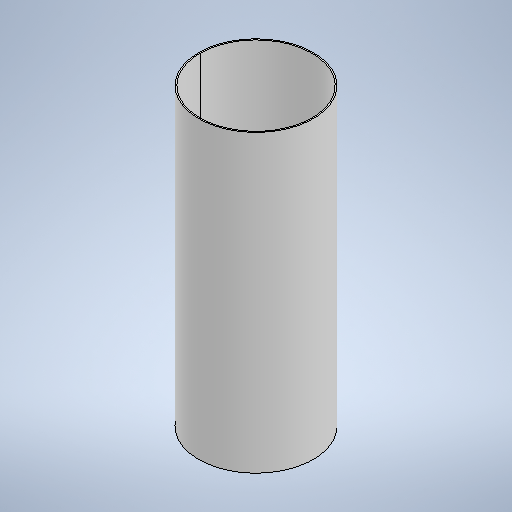
# Autodesk Inventor part: TZS 1291 accses hatch shell
Saved by Autodesk Inventor 2025 (Build 290162010, 162A)
## iProperties
Created: 2025-02-12
Part Number: TZS 1291 accses hatch shell
Material: Steel
Document SubType Name: Sheet Metal
Designer: admin
Mass: 13177.4 g
Surface Area: 5813.4 cm^2
Volume: 1678.65 cm^3
Density: 7.85 g/cm^3
Flat Pattern Width: 136 cm
Flat Pattern Length: 163.719 cm
Flat Pattern Area: 22265.8 cm^2
Sheet Metal Rule: Default_mm
Sheet Metal Width: 1360,000 mm
Sheet Metal Length: 1637,195 mm
Sheet Metal Area: 2226584,542 mm^2
Appearance: Default
Author: pokla
Autodesk Inventor part; units mm, degrees
ref_plane "YZ Plane" through (0, 0, 0) normal (1, 0, 0) x (0, 1, 0)
ref_plane "XZ Plane" through (0, 0, 0) normal (0, 1, 0) x (-1, 0, 0)
ref_plane "XY Plane" through (0, 0, 0) normal (0, 0, 1) x (1, 0, 0)
sketch "Sketch1" plane through (0, 0, 0) normal (0, 1, 0) x (-1, 0, 0)
  line L0 (258, 1360) -> (258, 0)
  line L1 (258, 0) -> (264, 0)
  line L2 (0, 0) -> (0, 109.131)
  line L3 (258, 1360) -> (264, 1360)
  line L4 (264, 0) -> (264, 1360)
  line L5 (263, 0) -> (259, 0)
  point P0 (261, 0)
  dimension "d3" = 6
  dimension "d5" = 1360
  dimension "d12" = 528
  constraints: 12 end point, 2 horizontal, 2 midpoint, 2 vertical, 1 horizontal alignment, 1 perpendicular
  measures "d3" distance of L0.end L1.end
  measures "d5" distance between parallel lines of L1 L3
  measures "d12" diameter of L4 L2
revolve "Revolution1" add sketch "Sketch1" angle 359.9 about axis through (0, 0, 0) along (0, 0, 1)
sketch "Sketch2" plane through (0, 0, 0) normal (0, 1, 0) x (-1, 0, 0)
  circle A0 centre (0, -706) radius 706
  point P0 (0, 0)
  dimension "d9" = 1412
  constraints: 2 vertical alignment, 2 other
extrude "Extrusion1" [suppressed]
equation "\"BendRadius\" = Thickness"
equation "\"BendReliefWidth\" = Thickness"
equation "\"BendReliefDepth\" = 0.5 * Thickness"
equation "\"CornerReliefSize\" = 4 * Thickness"
equation "\"MinimumRemnant\" = 2 * Thickness"
equation "\"TransitionRadius\" = BendRadius"
equation "\"JacobiRadiusSize\" = BendRadius"
equation "\"GapSize\" = Thickness"
equation "\"Thickness\" = 6"
body "Solid1"
